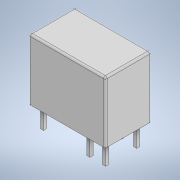
# Autodesk Inventor part: NRP03K
Saved by Autodesk Inventor 2021.2 (Build 252289000, 289)
## iProperties
Created: 2021-10-05
Part Number: NRP03K
Material: Типовые
Document SubType Name: Modeling
Designer: Kolan
Density: 1 g/cm^3
Appearance: По умолчанию
Author: Kolan
Autodesk Inventor part; units mm, degrees
ref_plane "YZ Plane" through (0, 0, 0) normal (1, 0, 0) x (0, 1, 0)
ref_plane "XZ Plane" through (0, 0, 0) normal (0, 1, 0) x (-1, 0, 0)
ref_plane "XY Plane" through (0, 0, 0) normal (0, 0, 1) x (1, 0, 0)
sketch "Эскиз1" plane through (0, 0, 0) normal (0, 1, 0) x (-1, 0, 0)
  line L0 (0, 0) -> (12.5, 0)
  line L1 (12.5, 0) -> (12.5, 7.5)
  line L2 (12.5, 7.5) -> (0, 7.5)
  line L3 (0, 7.5) -> (0, 0)
  dimension "d0" = 12.5
  dimension "d1" = 7.5
  constraints: 8 end point, 2 parallel, 1 horizontal, 1 perpendicular
  measures "d0" distance of L2.end L1.end
  measures "d1" distance of L1.end L0.end
extrude "Выдавливание1" add sketch "Эскиз1" along normal blind 10
sketch "Эскиз2" plane through (0, 0, 0) normal (0, -1, 0) x (1, 0, 0)
  line L0 (-1.42, 0.96) -> (-0.92, 0.96)
  line L1 (-0.92, 0.96) -> (-0.92, 1.46)
  line L2 (-0.92, 1.46) -> (-1.42, 1.46)
  line L3 (-1.42, 1.46) -> (-1.42, 0.96)
  line L4 (0, 0) -> (-12.5, 0) projected
  line L5 (0, 7.5) -> (0, 0) projected
  line L6 (-3.96, 0.96) -> (-3.46, 0.96)
  line L7 (-3.46, 0.96) -> (-3.46, 1.46)
  line L8 (-3.46, 1.46) -> (-3.96, 1.46)
  line L9 (-3.96, 1.46) -> (-3.96, 0.96)
  line L10 (-1.42, 6.04) -> (-0.92, 6.04)
  line L11 (-0.92, 6.04) -> (-0.92, 6.54)
  line L12 (-0.92, 6.54) -> (-1.42, 6.54)
  line L13 (-1.42, 6.54) -> (-1.42, 6.04)
  line L14 (-3.96, 6.04) -> (-3.46, 6.04)
  line L15 (-3.46, 6.04) -> (-3.46, 6.54)
  line L16 (-3.46, 6.54) -> (-3.96, 6.54)
  line L17 (-3.96, 6.54) -> (-3.96, 6.04)
  line L18 (-11.58, 6.04) -> (-11.08, 6.04)
  line L19 (-11.08, 6.54) -> (-11.58, 6.54)
  line L20 (-11.58, 6.54) -> (-11.58, 6.04)
  line L21 (-11.08, 6.04) -> (-11.08, 6.54)
  line L22 (-11.08, 1.46) -> (-11.58, 1.46)
  line L23 (-11.08, 0.96) -> (-11.08, 1.46)
  line L24 (-11.58, 1.46) -> (-11.58, 0.96)
  line L25 (-11.58, 0.96) -> (-11.08, 0.96)
  dimension "d4" = 0.5
  dimension "d5" = 0.5
  dimension "d7" = 0.96
  dimension "d8" = 0.92
  dimension "d11" = 2.54
  dimension "d14" = 5.08
  dimension "d19" = 7.62
  constraints: 48 end point, 3 horizontal, 2 parallel, 1 perpendicular, 1 vertical, 40 other
  measures "d4" distance of L2.end L1.end
  measures "d5" distance of L1.end L0.end
  measures "d7" distance between parallel lines of L4 L0
  measures "d8" distance between parallel lines of L5 L1
  measures "d11" distance of L0.start L6.start
  measures "d14" distance of L0.start L10.start
  measures "d19" distance of L14.start L18.start
extrude "Выдавливание2" add sketch "Эскиз2" along normal blind 3.5
fillet "Сопряжение1" radius 0.3 8 edges at (-6.25, 10, 0) (-12.5, 10, 3.75) (-6.25, 10, 7.5) (0, 10, 3.75) (0, 5, 7.5) (0, 5, 0) (-12.5, 5, 0) (-12.5, 5, 7.5)
